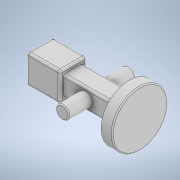
# Autodesk Inventor part: New_ThinGripper_base
Saved by Autodesk Inventor 2021 (Build 250183000, 183)
## iProperties
Created: 2021-08-05
Part Number: New_ThinGripper_base
Material: Generic
Document SubType Name: Modeling
Designer: hp
Density: 1 g/cm^3
Appearance: Default
Author: hp
Autodesk Inventor part; units mm, degrees
ref_plane "YZ Plane" through (0, 0, 0) normal (1, 0, 0) x (0, 1, 0)
sketch "Sketch1" plane through (0, 0, 0) normal (0, 0, 1) x (1, 0, 0)
  circle A0 centre (0, 0) radius 0.6
  dimension "d0" = 1.2
  constraints: 1 centre point, 1 coincident
  measures "d0" diameter of A0
extrude "Extrusion1" add sketch "Sketch1" against normal mid plane 6
sketch "Sketch3" plane through (0, 0, 0) normal (0, 0, 1) x (1, 0, 0)
  line L0 (0, 0) -> (3, 0)
  line L1 (0, 0) -> (-2, 0)
  line L2 (-2, 0) -> (-2, 0.9)
  line L3 (3, 0) -> (3, -0.9)
  line L4 (-2, 0.9) -> (3, 0.9)
  line L5 (3, 0.9) -> (3, -0.9)
  line L6 (3, -0.9) -> (-2, -0.9)
  line L7 (-2, -0.9) -> (-2, 0.9)
  dimension "d4" = 3
  dimension "d5" = 2
  dimension "d6" = 0.9
  dimension "d7" = 0.9
  constraints: 16 end point, 3 horizontal, 2 parallel, 2 vertical, 1 perpendicular
  measures "d4" distance of L0.start L0.end
  measures "d5" distance of L0.start L1.end
  measures "d6" distance of L1.end L2.end
  measures "d7" distance of L0.end L3.end
extrude "Extrusion2" add sketch "Sketch3" along normal mid plane 1.8
fillet "Fillet1" radius 0.2 4 edges at (0.5, 0.9, 0.9) (0.5, -0.9, 0.9) (0.5, 0.9, -0.9) (0.5, -0.9, -0.9)
ref_plane "Work Plane1" through (3, -0.7, -0.9) normal (1, 0, 0) x (0, 0, -1)
sketch "Sketch4" plane through (3, -0.7, -0.9) normal (1, 0, 0) x (0, 0, -1)
  circle A0 centre (-0.9, 0.7) radius 2.5
  dimension "d12" = 5
  constraints: 1 centre point, 1 coincident
  measures "d12" diameter of A0
extrude "Extrusion3" add sketch "Sketch4" along normal blind 1
ref_plane "Work Plane2" through (-2, -0.7, 0.9) normal (-1, 0, 0) x (0, 0, 1)
sketch "Sketch5" plane through (-2, -0.7, 0.9) normal (-1, 0, 0) x (0, 0, 1)
  line L0 (-2.1, -0.6) -> (0.3, -0.6)
  line L1 (0.3, -0.6) -> (0.3, 2)
  line L2 (0.3, 2) -> (-2.1, 2)
  line L3 (-2.1, 2) -> (-2.1, -0.6)
  line L4 (-2.1, -0.6) -> (0.3, 2) construction
  line L5 (0.3, -0.6) -> (-2.1, 2) construction
  point P0 (-0.9, 0.7)
  dimension "d16" = 2.4
  dimension "d17" = 2.6
  constraints: 12 end point, 2 midpoint, 2 parallel, 1 horizontal, 1 perpendicular
  measures "d16" distance of L0.start L0.end
  measures "d17" distance of L1.end L0.end
extrude "Extrusion4" add sketch "Sketch5" along normal blind 3
fillet "Fillet2" radius 0.2 12 edges at (-2, -1.3, 0) (-3.5, -1.3, -1.2) (-2, 0, -1.2) (-5, 0, -1.2) (-5, -1.3, 0) (-3.5, -1.3, 1.2) (-5, 0, 1.2) (-5, 1.3, 0) (-3.5, 1.3, 1.2) (-3.5, 1.3, -1.2) (-2, 1.3, 0) (-2, 0, 1.2)
fillet "Fillet3" radius 0.1 3 edges at (4, 0, 2.5) (-0.6, 0, 3) (-0.6, 0, -3)
body "Solid1"
